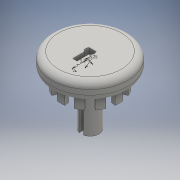
# Autodesk Inventor part: Wheel
Saved by Autodesk Inventor 2016 (Build 200138000, 138)
## iProperties
Created: 2015-06-04
Part Number: Wheel
Material: Generic
Document SubType Name: Modeling
Designer: Erin
Density: 1 g/cm^3
Appearance: Default
Author: Erin
Autodesk Inventor part; units mm, degrees
ref_plane "YZ Plane" through (0, 0, 0) normal (1, 0, 0) x (0, 1, 0)
ref_plane "XZ Plane" through (0, 0, 0) normal (0, 1, 0) x (-1, 0, 0)
ref_plane "XY Plane" through (0, 0, 0) normal (0, 0, 1) x (1, 0, 0)
sketch "Sketch1" plane through (0, 0, 0) normal (0, 0, 1) x (1, 0, 0)
  circle A0 centre (0, 0) radius 17.5
  dimension "d0" = 35
  constraints: 1 centre point, 1 coincident
  measures "d0" diameter of A0
extrude "Extrusion1" add sketch "Sketch1" against normal blind 4.15
sketch "Sketch2" plane through (0, 0, -4.15) normal (0, 0, -1) x (-1, 0, 0)
  circle A0 centre (0, 0) radius 13.5
  circle A1 centre (0, 0) radius 11.5
  circle A2 centre (0, 0) radius 17.5 projected
  circle A3 centre (0, 0) radius 17.5
  line L0 (0, 0) -> (-1.5011, 11.4016)
  line L1 (0, 0) -> (1.5011, 11.4016)
  line L2 (1.9711, 14.9723) -> (-1.9711, 14.9723)
  line L3 (-1.0506, 7.9799) -> (1.0506, 7.9799)
  line L4 (0, 0) -> (0, 14.9723) construction
  line L5 (-18.7051, 0) -> (19.1396, 0) construction
  line L6 (-1.5011, 11.4016) -> (-1.7621, 13.3845)
  line L7 (-1.7621, 13.3845) -> (-1.9711, 14.9723)
  line L8 (1.5011, 11.4016) -> (1.7621, 13.3845)
  line L9 (1.7621, 13.3845) -> (1.9711, 14.9723)
  dimension "d3" = 27
  dimension "d4" = 2
  dimension "d7" = 15
  constraints: 20 end point, 4 horizontal, 4 point on circle, 3 centre point, 3 coincident, 2 point on line, 1 concentric, 1 midpoint, 1 perpendicular
  measures "d3" diameter of A0
  measures "d4" radial gap between concentric circles of A1 A0
  measures "d7" angle of L1 L0
extrude "Extrusion2" add sketch "Sketch2" along normal blind 4.15 contours A0 L7 L2 L9 | A2
extrude "Extrusion3" add sketch "Sketch2" along normal blind 10 contours L8 A1 L6 A0 picked at (-0.1672, 12.8211)
extrude "Extrusion4" add sketch "Sketch2" along normal blind 2 contours A0 L6 A1 L8 | L8 A1 L6 A0
pattern_circular "Circular Pattern1" count 12 over 360 about axis through (0, 0, -10) along (0, 0, 1) of "Extrusion3"
fillet "Fillet1" radius 3 2 edges at (17.5, 0, -8.3) (-17.5, 0, 0)
sketch "Sketch3" plane through (0, 0, -4.15) normal (0, 0, -1) x (-1, 0, 0)
  circle A0 centre (0, 0) radius 4.125
  arc A1 (-1.6, 1.2) -> (1.6, 1.2) centre (0, 0) ccw
  line L0 (-1.6, 1.2) -> (1.6, 1.2)
  line L1 (-1.8267, -2) -> (2.2601, -2) construction
  line L2 (-1, 0) -> (1, 0)
  line L3 (1, 0) -> (1, -7)
  line L4 (1, -7) -> (-1, -7)
  line L5 (-1, -7) -> (-1, 0)
  arc A2 (1.6, 1.2) -> (-1.6, 1.2) centre (0, 0) ccw
  dimension "d16" = 8.25
  dimension "d17" = 4
  dimension "d18" = 3.2
  dimension "d19" = 2
  dimension "d20" = 7
  constraints: 12 end point, 4 point on circle, 3 centre point, 3 coincident, 3 horizontal, 2 midpoint, 2 parallel, 1 perpendicular, 1 tangent
  measures "d16" diameter of A0
  measures "d17" diameter of A1
  measures "d18" distance between parallel lines of L1 L0
  measures "d19" distance of L3.end L4.end
  measures "d20" distance of L2.end L3.end
extrude "Extrusion5" add sketch "Sketch3" along normal blind 27 contours A0 L3 A1 A2 L5 | L5 A1 L3 A0 | L5 L2 L3 A1 | A1 L0 L3 L2 L5 | A2 L0
extrude "Extrusion6" cut sketch "Sketch3" along normal mid plane 54 contours L5 A1 L3 A0 | A0 L3 L4 L5 | L5 L2 L3 A1 | A1 L0 L3 L2 L5
body "Solid1"
